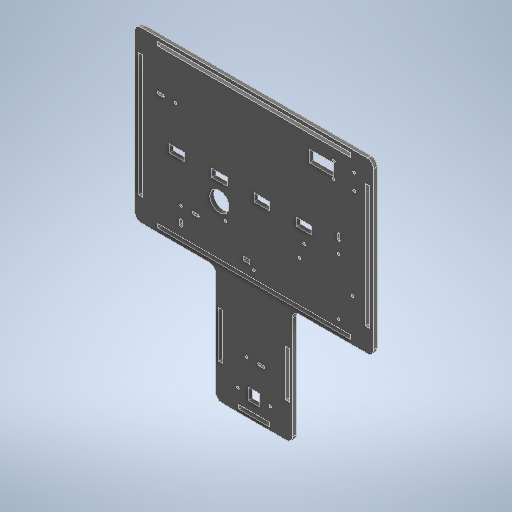
# Autodesk Inventor part: Sorting Mechanism Base Fixation
Saved by Autodesk Inventor 2025.4 (Build 294407000, 407)
## iProperties
Created: 2026-03-21
Part Number: Sorting Mechanism Base Fixation
Material: Generic
Document SubType Name: Sheet Metal
Designer: lenovo
Density: 1 g/cm^3
Sheet Metal Rule: Default_mm
Appearance: Gray
Author: lenovo
Autodesk Inventor part; units mm, degrees
ref_plane "YZ Plane" through (0, 0, 0) normal (1, 0, 0) x (0, 1, 0)
ref_plane "XZ Plane" through (0, 0, 0) normal (0, 1, 0) x (-1, 0, 0)
ref_plane "XY Plane" through (0, 0, 0) normal (0, 0, 1) x (1, 0, 0)
sketch "Sketch1" plane through (0, 0, 0) normal (0, 0, 1) x (1, 0, 0)
  line L0 (-155, 110) -> (155, 110)
  line L1 (155, 110) -> (155, -110)
  line L2 (155, -110) -> (-155, -110)
  line L3 (-155, -110) -> (-155, 110)
  line L4 (-155, 110) -> (155, -110) construction
  line L5 (155, 110) -> (-155, -110) construction
  circle A0 centre (130, 64.5) radius 1.65
  circle A1 centre (130, 85) radius 1.65
  circle A2 centre (103.5, 85) radius 1.65
  circle A3 centre (103.5, 64.5) radius 1.65
  circle A4 centre (-0.25, -89.75) radius 1.65
  circle A5 centre (-102.25, 47.25) radius 1.65
  line L6 (-13.75, -80.75) -> (-5.75, -80.75)
  line L7 (-5.75, -80.75) -> (-5.75, -85.75)
  line L8 (-5.75, -85.75) -> (-13.75, -85.75)
  line L9 (-13.75, -85.75) -> (-13.75, -80.75)
  line L10 (-13.75, -80.75) -> (-5.75, -85.75) construction
  line L11 (-5.75, -80.75) -> (-13.75, -85.75) construction
  line L12 (103.5, 67.25) -> (72, 67.25)
  line L13 (72, 67.25) -> (72, 82.25)
  line L14 (72, 82.25) -> (103.5, 82.25)
  line L15 (103.5, 82.25) -> (103.5, 67.25)
  line L16 (103.5, 67.25) -> (72, 82.25) construction
  line L17 (72, 67.25) -> (103.5, 82.25) construction
  circle A6 centre (-45, -35) radius 12.5
  point P0 (0, 0)
  point P1 (-9.75, -83.25)
  point P2 (87.75, 74.75)
  point P3 (103.5, 74.75)
  dimension "d0" = 310
  dimension "d1" = 220
  dimension "d2" = 3.3
  dimension "d4" = 20.5
  dimension "d7" = 3.3
  dimension "d8" = 25
  dimension "d9" = 25
  dimension "d10" = 26.5
  dimension "d11" = 3.3
  dimension "d12" = 205.75
  dimension "d13" = 17.25
  dimension "d14" = 154.25
  dimension "d15" = 103.75
  dimension "d16" = 4
  dimension "d17" = 5.5
  dimension "d18" = 8
  dimension "d19" = 5
  dimension "d21" = 10.25
  dimension "d22" = 31.5
  dimension "d23" = 15
  dimension "d24" = 25
  dimension "d27" = 75
  dimension "d28" = 110
  measures "d0" distance of L0.start L0.end
  measures "d1" distance of L2.end L0.start
  measures "d2" diameter of A0
  measures "d4" distance of A1.centre A0.centre
  measures "d7" diameter of A4
  measures "d8" distance from line of L0 A1.centre
  measures "d9" distance from line of L1 A1.centre
  measures "d10" distance of A1.centre A2.centre
  measures "d11" diameter of A5
  measures "d12" horizontal distance of A3.centre A5.centre
  measures "d13" vertical distance of A5.centre A3.centre
  measures "d14" vertical distance of A4.centre A3.centre
  measures "d15" horizontal distance of A4.centre A3.centre
  measures "d16" vertical distance of L7.end A4.centre
  measures "d17" distance from line of L7 A4.centre
  measures "d18" distance of L6.start L6.end
  measures "d19" distance of L8.end L6.start
  measures "d21" distance of point (103.5, 74.75) A2.centre
  measures "d22" distance of L13.end L14.end
  measures "d23" distance of L12.end L13.end
  measures "d24" diameter of A6
  measures "d27" distance from line of L2 A6.centre
  measures "d28" distance from line of L3 A6.centre
extrude "Plate1" add sketch "Sketch1" along normal blind 5
sketch "Sketch6" plane through (0, 0, 5) normal (0, 0, 1) x (1, 0, 0)
  line L0 (144.9, 80) -> (150, 80)
  line L1 (150, 80) -> (150, -80)
  line L2 (150, -80) -> (144.9, -80)
  line L3 (144.9, -80) -> (144.9, 80)
  line L4 (-125, 99.9) -> (125, 99.9)
  line L5 (125, 99.9) -> (125, 105)
  line L6 (125, 105) -> (-125, 105)
  line L7 (-125, 105) -> (-125, 99.9)
  line L8 (155, 110) -> (155, -110) projected
  line L9 (-155, 110) -> (155, 110) projected
  point P0 (0, 0)
  point P1 (144.9, 0)
  point P2 (155, 0)
  point P3 (0, 105)
  point P4 (0, 110)
  dimension "d53" = 160
  dimension "d54" = 5.1
  dimension "d55" = 5
  dimension "d56" = 5.1
  dimension "d57" = 5
  dimension "d58" = 250
  constraints: 16 end point, 4 midpoint, 4 parallel, 2 horizontal, 2 perpendicular, 1 horizontal alignment, 1 vertical alignment
  measures "d53" distance of L0.end L1.end
  measures "d54" distance of L0.start L0.end
  measures "d55" distance between parallel lines of L8 L1
  measures "d56" distance of L6.end L4.start
  measures "d57" distance between parallel lines of L9 L6
  measures "d58" distance of L5.end L6.end
extrude "Cut4" cut sketch "Sketch6" against normal blind 5
mirror "Mirror1" about plane through (0, 0, 0) normal (0, 1, 0) of "Cut4"
mirror "Mirror2" about plane through (0, 0, 0) normal (1, 0, 0) of "Cut4"
sketch "Sketch7" plane through (0, 0, 0) normal (0, 0, -1) x (-1, 0, 0)
  line L0 (50, -110) -> (-50, -110)
  line L1 (-50, -110) -> (-50, -260)
  line L2 (-50, -260) -> (50, -260)
  line L3 (50, -260) -> (50, -110)
  line L4 (155, -110) -> (-155, -110)
  line L5 (7.5, -240) -> (-7.5, -240)
  line L6 (-7.5, -240) -> (-7.5, -225)
  line L7 (-7.5, -225) -> (7.5, -225)
  line L8 (7.5, -225) -> (7.5, -240)
  line L9 (0, -240) -> (0, -225)
  circle A0 centre (-21, -232.5) radius 1.65
  circle A1 centre (21, -232.5) radius 1.65
  point P0 (0, 0)
  point P1 (0, -260)
  point P2 (0, -110)
  point P3 (0, -110)
  point P4 (0, -232.5)
  dimension "d61" = 100
  dimension "d62" = 150
  dimension "d68" = 15
  dimension "d69" = 20
  dimension "d70" = 3.3
  dimension "d71" = 42
  measures "d61" distance of L1.end L2.end
  measures "d62" distance of L0.end L1.end
  measures "d68" distance of L5.end L6.end
  measures "d69" distance between parallel lines of L2 L5
  measures "d70" diameter of A0
  measures "d71" diameter of A0.centre L9
sheet face with bend "Path Extension" sketch "Sketch7" thickness 5 toward (0, 0, 1) bend radius 5
bend "Bend1"
sketch "Sketch8" plane through (0, 0, 0) normal (0, 0, -1) x (-1, 0, 0)
  line L0 (20, -256) -> (-20, -256)
  line L1 (-20, -256) -> (-20, -250.8)
  line L2 (-20, -250.8) -> (20, -250.8)
  line L3 (20, -250.8) -> (20, -256)
  line L4 (20, -256) -> (-20, -250.8) construction
  line L5 (-20, -256) -> (20, -250.8) construction
  line L6 (-50, -260) -> (50, -260) projected
  line L7 (-7.5, -240) -> (7.5, -240) projected
  line L8 (0, -240) -> (0, -225)
  line L9 (-7.5, -225) -> (7.5, -225) projected
  line L10 (46, -155) -> (40.8, -155)
  line L11 (40.8, -155) -> (40.8, -215)
  line L12 (40.8, -215) -> (46, -215)
  line L13 (46, -215) -> (46, -155)
  line L14 (46, -155) -> (40.8, -215) construction
  line L15 (40.8, -155) -> (46, -215) construction
  line L16 (50, -260) -> (50, -110) projected
  line L17 (-46, -155) -> (-40.8, -155)
  line L18 (-40.8, -155) -> (-40.8, -215)
  line L19 (-40.8, -215) -> (-46, -215)
  line L20 (-46, -215) -> (-46, -155)
  line L21 (-46, -155) -> (-40.8, -215) construction
  line L22 (-40.8, -155) -> (-46, -215) construction
  point P0 (0, 0)
  point P1 (0, -253.4)
  point P2 (0, -260)
  point P3 (43.4, -185)
  point P4 (46, -185)
  point P5 (50, -185)
  point P6 (-43.4, -185)
  point P7 (-46, -185)
  dimension "d72" = 40
  dimension "d73" = 5.2
  dimension "d74" = 4
  dimension "d75" = 5.2
  dimension "d76" = 4
  dimension "d77" = 60
  constraints: 38 end point, 9 midpoint, 6 symmetric about line, 4 parallel, 2 horizontal, 2 perpendicular, 1 horizontal alignment, 1 vertical alignment
  measures "d72" distance of L1.end L2.end
  measures "d73" distance of L0.end L1.end
  measures "d74" distance between parallel lines of L6 L0
  measures "d75" distance of L11.end L12.end
  measures "d76" distance between parallel lines of L16 L13
  measures "d77" distance of L10.end L11.end
extrude "Cut5" cut sketch "Sketch8" against normal blind 5
sketch "Sketch9" plane through (0, 0, 0) normal (0, 0, -1) x (-1, 0, 0)
  line L0 (-55, -12.75) -> (-75, -12.75)
  line L1 (-75, -12.75) -> (-75, -2.75)
  line L2 (-75, -2.75) -> (-55, -2.75)
  line L3 (-55, -2.75) -> (-55, -12.75)
  line L4 (-155, 110) -> (155, 110) projected
  line L5 (-155, -110) -> (-155, 110) projected
  line L6 (-20, -12.75) -> (0, -12.75)
  line L7 (0, -12.75) -> (0, -2.75)
  line L8 (0, -2.75) -> (-20, -2.75)
  line L9 (-20, -2.75) -> (-20, -12.75)
  line L10 (35, -12.75) -> (55, -12.75)
  line L11 (55, -12.75) -> (55, -2.75)
  line L12 (55, -2.75) -> (35, -2.75)
  line L13 (35, -2.75) -> (35, -12.75)
  line L14 (90, -12.75) -> (110, -12.75)
  line L15 (110, -12.75) -> (110, -2.75)
  line L16 (110, -2.75) -> (90, -2.75)
  line L17 (90, -2.75) -> (90, -12.75)
  point P0 (0, 0)
  point P1 (-55, -7.75)
  point P2 (-20, -7.75)
  point P3 (0, -7.75)
  point P4 (35, -7.75)
  point P5 (55, -7.75)
  point P6 (90, -7.75)
  dimension "d80" = 10
  dimension "d81" = 20
  dimension "d82" = 112.75
  dimension "d83" = 80
  dimension "d84" = 35
  dimension "d85" = 35
  dimension "d86" = 35
  constraints: 32 end point, 8 parallel, 6 equal length, 6 midpoint, 4 horizontal, 4 perpendicular, 3 horizontal alignment
  measures "d80" distance of L0.end L1.end
  measures "d81" distance of L0.start L0.end
  measures "d82" distance between parallel lines of L4 L2
  measures "d83" distance between parallel lines of L5 L1
  measures "d84" distance between parallel lines of L3 L9
  measures "d85" distance between parallel lines of L13 L7
  measures "d86" distance between parallel lines of L17 L11
extrude "Cut6" cut sketch "Sketch9" against normal blind 5
sketch "Sketch10" plane through (0, 0, 5) normal (0, 0, 1) x (1, 0, 0)
  circle A0 centre (-37.25, -52.75) radius 1.6
  circle A1 centre (-0.25, -89.75) radius 1.65 projected
  circle A2 centre (110, -89.75) radius 1.6
  circle A3 centre (59, -46.55) radius 1.6
  line L0 (125, -99.9) -> (125, -105) projected
  circle A4 centre (-94.9, -64.9) radius 1.6
  line L1 (-125, -99.9) -> (125, -99.9) projected
  line L2 (-144.9, 80) -> (-144.9, -80) projected
  line L3 (-78.9, -64.9) -> (-72.9, -64.9) construction
  line L4 (-78.9, -66.5) -> (-72.9, -66.5)
  line L5 (-72.9, -63.3) -> (-78.9, -63.3)
  arc A5 (-78.9, -63.3) -> (-78.9, -66.5) centre (-78.9, -64.9) ccw
  arc A6 (-72.9, -66.5) -> (-72.9, -63.3) centre (-72.9, -64.9) ccw
  point P0 (0, 0)
  point P1 (-75.9, -64.9)
  dimension "d89" = 3.2
  dimension "d91" = 37
  dimension "d92" = 3.2
  dimension "d93" = 3.2
  dimension "d94" = 43.2
  dimension "d95" = 51
  dimension "d96" = 15
  dimension "d98" = 37
  dimension "d101" = 3.2
  dimension "d102" = 35
  dimension "d103" = 50
  dimension "d112" = 1.6
  dimension "d113" = 6
  dimension "d114" = 19
  constraints: 8 end point, 6 centre point, 4 point on circle, 4 tangent, 2 horizontal alignment, 1 horizontal, 1 midpoint, 1 parallel
  measures "d89" diameter of A0
  measures "d91" horizontal distance of A1.centre A0.centre
  measures "d92" diameter of A2
  measures "d93" diameter of A3
  measures "d94" vertical distance of A3.centre A2.centre
  measures "d95" horizontal distance of A2.centre A3.centre
  measures "d96" distance from line of L0 A2.centre
  measures "d98" horizontal distance of A0.centre A1.centre
  measures "d101" diameter of A4
  measures "d102" distance from line of L1 A4.centre
  measures "d103" distance from line of L2 A4.centre
  measures "d112" radius of A6
  measures "d113" distance of L3.start L3.end
  measures "d114" distance of A4.centre point (-75.9, -64.9)
extrude "Cut7" cut sketch "Sketch10" against normal blind 5 contours A0 | A2 | A3 | A4 | A5 L5 A6 L4
sketch "Sketch11" plane through (0, 0, 0) normal (0, 0, -1) x (-1, 0, 0)
  line L0 (118.25, 47.25) -> (124.25, 47.25) construction
  line L1 (118.25, 45.65) -> (124.25, 45.65)
  line L2 (124.25, 48.85) -> (118.25, 48.85)
  arc A0 (118.25, 48.85) -> (118.25, 45.65) centre (118.25, 47.25) ccw
  arc A1 (124.25, 45.65) -> (124.25, 48.85) centre (124.25, 47.25) ccw
  circle A2 centre (102.25, 47.25) radius 1.65 projected
  point P0 (0, 0)
  point P1 (121.25, 47.25)
  dimension "d106" = 1.6
  dimension "d108" = 19
  dimension "d109" = 6
  constraints: 8 end point, 4 point on circle, 4 tangent, 2 centre point, 1 horizontal, 1 horizontal alignment, 1 midpoint, 1 parallel
  measures "d106" radius of A1
  measures "d108" distance of A2.centre point (121.25, 47.25)
  measures "d109" distance of L0.start L0.end
extrude "Cut8" cut sketch "Sketch11" against normal blind 5 contours A0 L2 A1 L1
sketch "Sketch12" plane through (0, 0, 5) normal (0, 0, 1) x (1, 0, 0)
  circle A0 centre (-9.5, -192.5) radius 1.6
  line L0 (6.5, -192.5) -> (12.5, -192.5) construction
  line L1 (6.5, -194.1) -> (12.5, -194.1)
  line L2 (12.5, -190.9) -> (6.5, -190.9)
  arc A1 (6.5, -190.9) -> (6.5, -194.1) centre (6.5, -192.5) ccw
  arc A2 (12.5, -194.1) -> (12.5, -190.9) centre (12.5, -192.5) ccw
  line L3 (7.5, -225) -> (-7.5, -225) projected
  line L4 (0, -225) -> (0, -105)
  line L5 (125, -105) -> (-125, -105) projected
  circle A3 centre (-21, -232.5) radius 1.65 projected
  line L6 (-94.9, -86.9) -> (-94.9, -80.9) construction
  line L7 (-93.3, -86.9) -> (-93.3, -80.9)
  line L8 (-96.5, -80.9) -> (-96.5, -86.9)
  arc A4 (-96.5, -86.9) -> (-93.3, -86.9) centre (-94.9, -86.9) ccw
  arc A5 (-93.3, -80.9) -> (-96.5, -80.9) centre (-94.9, -80.9) ccw
  circle A6 centre (-94.9, -64.9) radius 1.6 projected
  point P0 (0, 0)
  point P1 (9.5, -192.5)
  point P2 (-94.9, -83.9)
  dimension "d115" = 3.2
  dimension "d116" = 1.6
  dimension "d117" = 6
  dimension "d118" = 19
  dimension "d119" = 40
  dimension "d122" = 6
  dimension "d123" = 19
  constraints: 18 end point, 8 point on circle, 8 tangent, 5 centre point, 4 midpoint, 2 parallel, 1 equal radius, 1 horizontal, 1 horizontal alignment, 1 symmetric about line, 1 vertical, 1 vertical alignment
  measures "d115" diameter of A0
  measures "d116" radius of A2
  measures "d117" distance of L0.start L0.end
  measures "d118" distance of point (9.5, -192.5) A0.centre
  measures "d119" vertical distance of A3.centre A0.centre
  measures "d122" distance of L6.start L6.end
  measures "d123" distance of point (-94.9, -83.9) A6.centre
extrude "Cut9" cut sketch "Sketch12" against normal blind 5 contours A0 | A1 L2 A2 L1 | A4 L8 A5 L7
sketch "Sketch13" plane through (0, 0, 5) normal (0, 0, 1) x (1, 0, 0)
  circle A0 centre (109.9, -16.55) radius 1.6
  line L0 (109.9, -0.55) -> (109.9, 5.45) construction
  line L1 (111.5, -0.55) -> (111.5, 5.45)
  line L2 (108.3, 5.45) -> (108.3, -0.55)
  arc A1 (108.3, -0.55) -> (111.5, -0.55) centre (109.9, -0.55) ccw
  arc A2 (111.5, 5.45) -> (108.3, 5.45) centre (109.9, 5.45) ccw
  line L3 (144.9, 80) -> (144.9, -80) projected
  line L4 (144.9, 0) -> (0, 0)
  line L5 (144.9, -80) -> (144.9, 80) projected
  circle A3 centre (59, -46.55) radius 1.6 projected
  point P0 (109.9, 2.45)
  dimension "d124" = 3.2
  dimension "d125" = 6
  dimension "d126" = 19
  dimension "d127" = 35
  dimension "d130" = 30
  constraints: 10 end point, 4 point on circle, 4 tangent, 3 centre point, 3 midpoint, 1 equal radius, 1 horizontal, 1 parallel, 1 vertical, 1 vertical alignment
  measures "d124" diameter of A0
  measures "d125" distance of L0.start L0.end
  measures "d126" distance of point (109.9, 2.45) A0.centre
  measures "d127" horizontal distance of point (144.9, 0) A0.centre
  measures "d130" vertical distance of A3.centre A0.centre
extrude "Cut10" cut sketch "Sketch13" against normal blind 5 contours A0 | A1 L2 L4 L1 | L4 L2 A2 L1
sketch "Sketch14" plane through (0, 0, 5) normal (0, 0, 1) x (1, 0, 0)
  circle A0 centre (128, -54.75) radius 1.6
  circle A1 centre (110, -89.75) radius 1.6 projected
  circle A2 centre (65, -27.75) radius 1.6
  line L0 (75, -12.75) -> (55, -12.75) projected
  point P0 (0, 0)
  point P1 (65, -12.75)
  dimension "d131" = 3.2
  dimension "d132" = 35
  dimension "d133" = 18
  dimension "d136" = 3.2
  dimension "d137" = 15
  constraints: 2 centre point, 1 midpoint, 1 vertical alignment
  measures "d131" diameter of A0
  measures "d132" vertical distance of A0.centre A1.centre
  measures "d133" horizontal distance of A1.centre A0.centre
  measures "d136" diameter of A2
  measures "d137" distance from line of A2.centre L0
extrude "Cut11" cut sketch "Sketch14" against normal blind 5 contours A0 | A2
fillet "Corner Round1" radius 8 10 edges at (155, 110, 2.5) (155, -110, 2.5) (50, -110, 0.6699) (50, -110, 3.1699) (50, -260, 2.5) (-50, -260, 2.5) (-50, -110, 0.6699) (-50, -110, 3.1699) (-155, -110, 2.5) (-155, 110, 2.5)
equation "\"d59\" = Thickness"
equation "\"d75\" = d73"
equation "\"d76\" = d74"
equation "\"d78\" = Thickness"
equation "\"d87\" = Thickness"
equation "\"d99\" = Thickness"
equation "\"d110\" = Thickness"
equation "\"d120\" = Thickness"
equation "\"d128\" = Thickness"
equation "\"d134\" = Thickness"
equation "\"d20\" = Thickness"
equation "\"d63\" = BendRadius"
equation "\"d64\" = BendReliefWidth"
equation "\"d66\" = MinimumRemnant"
equation "\"d65\" = BendReliefDepth"
equation "\"d67\" = TransitionRadius"
equation "\"BendRadius\" = Thickness"
equation "\"BendReliefWidth\" = Thickness"
equation "\"BendReliefDepth\" = 0.5 * Thickness"
equation "\"TransitionRadius\" = BendRadius"
equation "\"JacobiRadiusSize\" = BendRadius"
equation "\"GapSize\" = Thickness"
equation "\"Thickness\" = 5"
equation "\"MinimumRemnant\" = 10"
body "Solid1"
